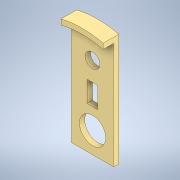
# Autodesk Inventor part: wheel_P1
Saved by Autodesk Inventor 2020.1 (Build 241239000, 239)
## iProperties
Created: 2020-01-18
Part Number: wheel_P1
Material: Generic
Document SubType Name: Modeling
Designer: Ali
Density: 1 g/cm^3
Appearance: Default
Author: Ali
Autodesk Inventor part; units mm, degrees
ref_plane "XY Plane" through (0, 0, 0) normal (0, 0, 1) x (1, 0, 0)
sketch "Sketch1" plane through (0, 0, 0) normal (0, 0, 1) x (1, 0, 0)
  circle A0 centre (0, 0) radius 36
  dimension "d0" = 72
  constraints: 1 centre point, 1 coincident
  measures "d0" diameter of A0
extrude "Extrusion1" add sketch "Sketch1" along normal blind 2
sketch "Sketch2" plane through (0, 0, 2) normal (0, 0, 1) x (1, 0, 0)
  circle A0 centre (0, 0) radius 36 projected
  circle A1 centre (0, 0) radius 34
  dimension "d3" = 2
  constraints: 1 centre point
  measures "d3" radial gap between concentric circles of A0 A1
extrude "Extrusion2" add sketch "Sketch2" along normal blind 4
sketch "Sketch4" plane through (0, 0, 2) normal (0, 0, 1) x (1, 0, 0)
  point P0 (0, 0)
  point P1 (0, 0)
  constraints: 1 coincident
hole "Hole1" at (0, 0, 2) direction (0, 0, -1) diameter 10.1 end through all
sketch "Sketch5" plane through (0, 0, 2) normal (0, 0, 1) x (1, 0, 0)
  point P0 (0, 0)
  point P1 (0, 23.3333)
  dimension "d13" = 23.3333
  measures "d13" distance of point (0, 0) point (0, 23.333)
hole "Hole2" at (0, 23.3333, 2) direction (0, 0, -1) diameter 5.6 end through all
pattern_circular "Circular Pattern1" count 5 over 360 about axis through (0, 0, -100) along (0, 0, 1) of "Hole2"
sketch "Sketch8" plane through (0, 0, 2) normal (0, 0, 1) x (1, 0, 0)
  circle A0 centre (22.1913, 7.2104) radius 2.8 projected
  circle A1 centre (13.715, -18.8771) radius 2.8 projected
  circle A2 centre (-13.715, -18.8771) radius 2.8 projected
  circle A3 centre (-22.1913, 7.2104) radius 2.8 projected
  circle A4 centre (0, 23.3333) radius 2.8 projected
  circle A5 centre (0, 0) radius 5.05 projected
  circle A6 centre (0, 0) radius 34 projected
  line L0 (-2, 16) -> (2, 16)
  line L1 (2, 16) -> (2, 8)
  line L2 (2, 8) -> (-2, 8)
  line L3 (-2, 8) -> (-2, 16)
  dimension "d43" = 4
  dimension "d44" = 8
  dimension "d45" = 8
  dimension "d48" = 2
  constraints: 8 end point, 2 parallel, 1 horizontal, 1 perpendicular
  measures "d43" distance of L0.start L0.end
  measures "d44" distance of L2.end L0.start
  measures "d45" distance from line of point (0, 0) L2
  measures "d48" distance from line of point (0, 0) L3
extrude "Extrusion5" cut sketch "Sketch8" against normal up to surface (2 mm away) contours L0 L1 L2 L3
ref_plane "Work Plane1" through (8.08, 0, 0) normal (1, 0, 0) x (0, 1, 0)
ref_plane "Work Plane2" through (-8.08, 0, 0) normal (1, 0, 0) x (0, 1, 0)
ref_plane "Work Plane3" through (0, -8.08, 0) normal (0, 1, 0) x (-1, 0, 0)
split "Split1" plane through (0, -8.08, 0) removes the side toward (0, -1, 0)
split "Split2" plane through (-8.08, 0, 0) removes the side toward (-1, 0, 0)
split "Split3" plane through (8.08, 0, 0) removes the side toward (1, 0, 0)
equation "\"d0\" = W_innerDiameter + W_wallThickness"
equation "\"d1\" = W_wallThickness"
equation "\"d3\" = W_wallThickness"
equation "\"d4\" = W_innerDepth"
equation "\"d6\" = W_innerGearHoleDiameter"
equation "\"d13\" = OG_distanceFromCenter"
equation "\"d14\" = W_outerGearHoleDiameter"
equation "\"W_wallThickness\" = 2"
equation "\"W_innerDepth\" = 4"
equation "\"W_innerGearHoleDiameter\" = 10.1"
equation "\"W_outerGearHoleDiameter\" = 5.6"
equation "\"OG_distanceFromCenter\" = 23.33333"
equation "\"W_innerDiameter\" = 70"
equation "\"Wheel_Related_W_\" = 0"
equation "\"W_holesClearance\" = 0.3"
equation "\"TempSpotReserved7\" = 0"
equation "\"TempSpotReserved8\" = 0"
equation "\"TempSpotReserved9\" = 0"
equation "\"TempSpotReserved10\" = 0"
equation "\"TempSpotReserved11\" = 0"
equation "\"TempSpotReserved12\" = 0"
equation "\"TempSpotReserved13\" = 0"
equation "\"TempSpotReserved14\" = 0"
equation "\"TempSpotReserved15\" = 0"
equation "\"TempSpotReserved16\" = 0"
equation "\"TempSpotReserved17\" = 0"
equation "\"TempSpotReserved18\" = 0"
equation "\"TempSpotReserved19\" = 0"
equation "\"TempSpotReserved20\" = 0"
equation "\"Inner_Gear_Related_IG_\" = 0"
equation "\"IG_shaftDiameter\" = 7.5"
equation "\"IG_shaftLength\" = 15"
equation "\"IG_gearThickness\" = 2"
equation "\"TempSpotReserved25\" = 0"
equation "\"TempSpotReserved26\" = 0"
equation "\"TempSpotReserved27\" = 0"
equation "\"TempSpotReserved28\" = 0"
equation "\"TempSpotReserved29\" = 0"
equation "\"TempSpotReserved30\" = 0"
equation "\"TempSpotReserved31\" = 0"
equation "\"TempSpotReserved32\" = 0"
equation "\"TempSpotReserved33\" = 0"
equation "\"TempSpotReserved34\" = 0"
equation "\"TempSpotReserved35\" = 0"
equation "\"TempSpotReserved36\" = 0"
equation "\"TempSpotReserved37\" = 0"
equation "\"TempSpotReserved38\" = 0"
equation "\"TempSpotReserved39\" = 0"
equation "\"TempSpotReserved40\" = 0"
equation "\"Outer_Gear_Related_OG_\" = 0"
equation "\"OG_shaftDiameter\" = 5"
equation "\"OG_gearDiameter\" = 26.66667"
equation "\"OG_shaftLength\" = 7"
equation "\"OG_gearThickness\" = 2"
equation "\"TempSpotReserved47\" = 0"
equation "\"TempSpotReserved48\" = 0"
equation "\"TempSpotReserved49\" = 0"
equation "\"TempSpotReserved50\" = 0"
equation "\"TempSpotReserved51\" = 0"
equation "\"TempSpotReserved52\" = 0"
equation "\"TempSpotReserved53\" = 0"
equation "\"TempSpotReserved54\" = 0"
equation "\"TempSpotReserved55\" = 0"
equation "\"TempSpotReserved56\" = 0"
equation "\"TempSpotReserved57\" = 0"
equation "\"TempSpotReserved58\" = 0"
equation "\"TempSpotReserved59\" = 0"
equation "\"TempSpotReserved60\" = 0"
equation "\"Leg_Extensions_Related_LE_\" = 0"
equation "\"LE_baseDiameter\" = 5"
equation "\"LE_maxLength\" = 24.6522"
equation "\"LE_thickness\" = 2.5"
equation "\"IG_ratioToOuterGear\" = 0.75"
equation "\"B_bearingThickness\" = 1"
equation "\"TempSpotReserved43\" = 0"
equation "\"TempSpotReserved45\" = 0"
equation "\"Thisisatest\" = 25.4"
equation "\"TempSpotReserved46\" = 0"
equation "\"TempSpotReserved44\" = 0"
equation "\"LE_offsetAboveOuterGear\" = 0"
equation "\"Bearing_Related_B_\" = 0"
equation "\"TempSpotReserved42\" = 0"
equation "\"OG_skirtOffset\" = 1"
equation "\"OG_skirtThickness\" = 1"
equation "\"IG_skirtThickness\" = 2"
equation "\"IG_extentionLength\" = 18.33333"
equation "\"IG_extentionThickness\" = 3"
equation "\"IG_slitWidth\" = 4"
equation "\"IG_slitlength\" = 8"
equation "\"IG_slitClearance\" = 0.15"
equation "\"IG_slitDistanceFromCenterHole\" = 8"
equation "\"Reserved_10\" = 0"
equation "\"Reserved_9\" = 0"
equation "\"Reserved_11\" = 0"
equation "\"Reserved_12\" = 0"
equation "\"Reserved_8\" = 0"
equation "\"Reserved_7\" = 0"
equation "\"Reserved_26\" = 0"
equation "\"Reserved_20\" = 0"
equation "\"Reserved_22\" = 0"
equation "\"Reserved_23\" = 0"
equation "\"Reserved_25\" = 0"
equation "\"Reserved_24\" = 0"
equation "\"Reserved_21\" = 0"
equation "\"Reserved_19\" = 0"
equation "\"Reserved_27\" = 0"
equation "\"Reserved_14\" = 0"
equation "\"Reserved_15\" = 0"
equation "\"Reserved_16\" = 0"
equation "\"Reserved_13\" = 0"
equation "\"Reserved_17\" = 0"
equation "\"Reserved_18\" = 0"
equation "\"Bearing_Related_BR_\" = 0"
equation "\"BR_bearingThickness\" = 1"
equation "\"Block_Related_BL_\" = 0"
equation "\"BL_width\" = 3.85"
equation "\"BL_length\" = 7.85"
body "Solid1"
